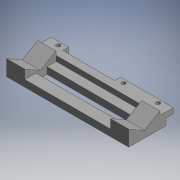
# Autodesk Inventor part: Base Extension 2
Saved by Autodesk Inventor 2020.5 (Build 245400000, 400)
## iProperties
Created: 2023-04-02
Part Number: Base Extension 2
Material: Generic
Document SubType Name: Modeling
Designer: Wes
Density: 1 g/cm^3
Appearance: Default
Author: Wes
Autodesk Inventor part; units mm, degrees
ref_plane "YZ Plane" through (0, 0, 0) normal (1, 0, 0) x (0, 1, 0)
ref_plane "XZ Plane" through (0, 0, 0) normal (0, 1, 0) x (-1, 0, 0)
ref_plane "XY Plane" through (0, 0, 0) normal (0, 0, 1) x (1, 0, 0)
sketch "Sketch1" plane through (0, 0, 0) normal (0, 0, 1) x (1, 0, 0)
  line L0 (0, 0) -> (0, 81.958)
  line L1 (0, 0) -> (0, -81.958)
  line L2 (0, -81.958) -> (-10, -81.958)
  line L3 (-5, -81.958) -> (-5, -67.708) construction
  line L4 (-5, -67.708) -> (-5, -58.708) construction
  line L5 (-10, -81.958) -> (-10, -58.708)
  line L6 (-10, -58.708) -> (0, -58.708)
  line L7 (0, 81.958) -> (-10, 81.958)
  line L8 (-5, 81.958) -> (-5, 66.21) construction
  line L9 (-5, 66.21) -> (-5, 20.031) construction
  line L10 (-5, 20.031) -> (-5, 11.031) construction
  line L11 (-10, 81.958) -> (-10, 11.031)
  line L12 (-10, 11.031) -> (0, 11.031)
  line L13 (0, -58.708) -> (-2, -58.708)
  line L14 (-2, -58.708) -> (-2, 11.031)
  line L15 (0, -81.958) -> (8, -81.958)
  line L16 (8, -81.958) -> (8, 81.958)
  line L17 (8, 81.958) -> (0, 81.958)
  line L18 (0, 81.958) -> (0, -81.958)
  dimension "d0" = 81.958
  dimension "d2" = 163.916
  dimension "d3" = 10
  dimension "d4" = 14.25
  dimension "d5" = 9
  dimension "d6" = 15.748
  dimension "d7" = 46.179
  dimension "d8" = 9
  dimension "d9" = 2
  dimension "d10" = 8
  constraints: 38 end point, 9 vertical, 4 perpendicular, 4 point on line, 3 horizontal, 2 midpoint, 2 parallel
  measures "d0" distance of L0.start L0.end
  measures "d2" distance of L1.end L0.end
  measures "d3" distance of L1.end L2.end
  measures "d4" distance of L3.start L3.end
  measures "d5" distance of L3.end L4.end
  measures "d6" distance of L8.start L8.end
  measures "d7" distance of L8.end L9.end
  measures "d8" distance of L9.end L10.end
  measures "d9" distance of L6.end L13.end
  measures "d10" distance of L17.end L16.end
extrude "Extrusion1" add sketch "Sketch1" along normal blind 7
sketch "Sketch2" plane through (0, 0, 0) normal (0, 0, -1) x (-1, 0, 0)
  line L0 (10, 81.958) -> (10, 11.031) construction
  line L1 (10, 46.4945) -> (0, 46.4945) construction
  line L2 (-8, 81.958) -> (10, 81.958) projected
  line L3 (0, 81.958) -> (-50, 81.958)
  line L4 (-50, 81.958) -> (-50, -81.958)
  line L5 (-50, -81.958) -> (0, -81.958)
  line L6 (0, -81.958) -> (0, 81.958)
  line L7 (-35.1508, -57.5) -> (-20.1508, -57.5)
  line L8 (-20.1508, -57.5) -> (-20.1508, 57.5)
  line L9 (-20.1508, 57.5) -> (-35.1508, 57.5)
  line L10 (-35.1508, 57.5) -> (-35.1508, -57.5)
  line L11 (-35.1508, -57.5) -> (-20.1508, 57.5) construction
  line L12 (-20.1508, -57.5) -> (-35.1508, 57.5) construction
  point P0 (0, 0)
  point P1 (-27.6508, 0)
  dimension "d13" = 10
  dimension "d14" = 50
  dimension "d15" = 15
  dimension "d16" = 115
  constraints: 22 end point, 4 parallel, 3 horizontal, 3 midpoint, 2 perpendicular, 1 point on line
  measures "d13" distance of L1.start L1.end
  measures "d14" distance of L5.end L4.end
  measures "d15" distance of L9.end L8.end
  measures "d16" distance of L8.end L7.end
extrude "Extrusion2" add sketch "Sketch2" along normal blind 9
sketch "Sketch3" plane through (-10, -81.958, 7) normal (0, -1, 0) x (1, 0, 0)
  line L0 (60, -7) -> (18, -7) projected
  line L1 (60, -7) -> (60, 5)
  line L2 (0, 0) -> (18, 0) projected
  line L3 (18, 5) -> (18, 0)
  line L4 (60, 5) -> (39, -7)
  line L5 (18, 5) -> (39, -7)
  line L6 (18, -7) -> (18, 0) projected
  line L7 (18, 0) -> (18, -7)
  point P0 (10, -7)
  dimension "d19" = 12
  constraints: 10 end point, 3 vertical, 1 midpoint
  measures "d19" distance of L0.start L1.end
extrude "Extrusion3" add sketch "Sketch3" against normal up to surface (24.458 mm away)
mirror "Mirror1" about plane through (0, 0, 0) normal (0, 1, 0) of "Extrusion3"
sketch "Sketch4" plane through (0, 0, 7) normal (0, 0, 1) x (1, 0, 0)
  line L0 (-5, -81.958) -> (-5, -67.708) construction
  line L1 (-5, 81.958) -> (-5, 66.21) construction
  line L2 (-5, 66.21) -> (-5, 20.031) construction
  circle A0 centre (-5, -67.708) radius 1.65
  circle A1 centre (-5, 20.031) radius 1.65
  circle A2 centre (-5, 66.21) radius 1.65
  point P0 (0, 0)
  dimension "d22" = 14.25
  dimension "d23" = 46.179
  dimension "d24" = 15.748
  dimension "d25" = 3.3
  constraints: 3 centre point, 3 coincident
  measures "d22" distance of L0.start L0.end
  measures "d23" distance of L1.end L2.end
  measures "d24" distance of L1.start L1.end
  measures "d25" diameter of A0
extrude "Extrusion4" cut sketch "Sketch4" against normal up to surface (7 mm away)
sketch "Sketch5" plane through (0, 0, 7) normal (0, 0, 1) x (1, 0, 0)
  circle A0 centre (-5, -67.708) radius 1.65 projected
  circle A1 centre (-5, -67.708) radius 2.65
  circle A2 centre (-5, 20.031) radius 1.65 projected
  circle A3 centre (-5, 20.031) radius 2.65
  circle A4 centre (-5, 66.21) radius 1.65 projected
  circle A5 centre (-5, 66.21) radius 2.65
  point P0 (0, 0)
  dimension "d28" = 5.3
  constraints: 3 centre point, 3 coincident
  measures "d28" diameter of A1
extrude "Extrusion5" cut sketch "Sketch5" against normal blind 6 contours A0 | A1 | A2 | A3 | A4 | A5
body "Solid1"
